Autodesk Fusion 360 part; units mm, degrees
(part 3 of 3)
ref_plane "WorkPlane14" through (0, 0, 17) normal (0, 0, 1) x (1, 0, 0)
sketch "Sketch18" plane through (0, 0, 17) normal (0, 0, 1) x (1, 0, 0)
  line L0 (575, 155) -> (300, 155)
  line L1 (575, 155) -> (575, 244.7658)
  line L2 (575, 244.7658) -> (300, 244.7658)
  line L3 (300, 244.7658) -> (300, 155)
  constraint horizontal L0
  constraint perpendicular L0 L1
  constraint perpendicular L1 L2
  constraint perpendicular L0 L3
extrude "Extrude17" cut sketch "Sketch18" against normal blind 200 bodies 6 7 8 9
extrude "Extrude18" add sketch "Sketch17" along normal mid plane 5 separate body makes body 13
mirror "Mirror2" about plane through (0, 0, 0) normal (1, 0, 0) of bodies 10 9 8 7 6 5 4 3 2 11 12 makes body 14 at (-72.5, 40.7662, 5.9313) makes body 15 at (-140, 40.7662, 5.9313) makes body 16 at (-211.5, 40.7662, 5.9313) makes body 17 at (-281.5, 40.7662, 5.9313) makes body 18 at (-351.5, 104.4646, 6.1744) makes body 19 at (-421.5, 104.4646, 6.1744) makes body 20 at (-491.5, 104.4646, 6.1744) makes body 21 at (-561.5, 104.4646, 6.1744) makes body 22 at (-600, 40.7662, 5.9313) makes body 23 at (-200, 62.2055, 10.1217) makes body 24 at (-200, 143.3882, 7.5489)
sketch "Sketch19" plane through (600, 0, 0) normal (1, 0, 0) x (0, 1, 0)
  spline S0 degree 3 poles (61.2364, 16.8866) (62.5517, 16.9377) (63.97, 16.9799) (65.4867, 17.0124) (69.0475, 17.0885) (73.1641, 17.1099) (77.299, 17.0516) (81.1898, 16.9968) (85.0421, 16.869) (88.6866, 16.6762) (93.5117, 16.421) (98.0281, 16.059) (102.6424, 15.6416) (107.4083, 15.2105) (112.3122, 14.7191) (117.3527, 14.1433) (123.7504, 13.4125) (130.3032, 12.5277) (136.4155, 11.5838) (140.28, 10.987) (143.9527, 10.3752) (147.6957, 9.7206) (151.3487, 9.0818) (155.1437, 8.3909) (159.2882, 7.6111) (162.7518, 6.9595) (166.4626, 6.2444) (170.0047, 5.5188) (173.5306, 4.7965) (176.8181, 4.0717) (179.5028, 3.4129) (180.7522, 3.1063) (181.8753, 2.8143) (182.9209, 2.533) knots 0 0 0 0 0.009474 0.009474 0.009474 0.031716 0.031716 0.031716 0.052644 0.052644 0.052644 0.080353 0.080353 0.080353 0.108972 0.108972 0.108972 0.145296 0.145296 0.145296 0.168261 0.168261 0.168261 0.190675 0.190675 0.190675 0.209405 0.209405 0.209405 0.22805 0.22805 0.22805 0.236727 0.236727 0.236727 0.236727
  spline S1 degree 3 poles (182.9209, 2.533) (181.6615, 2.4681) (180.2835, 2.4098) (178.7296, 2.3656) (175.4512, 2.2724) (171.3919, 2.2497) (167.2511, 2.2303) (163.72, 2.2137) (160.1948, 2.1893) (156.9225, 2.1285) (150.7153, 2.0131) (145.3748, 1.778) (139.6944, 1.5684) (135.7191, 1.4217) (131.5605, 1.2846) (127.3, 1.1404) (121.7528, 0.9526) (116.1156, 0.7389) (110.7376, 0.5168) (105.8624, 0.3155) (101.2103, 0.121) (96.4895, -0.064) (92.2873, -0.2286) (87.9529, -0.3939) (83.3434, -0.5864) (76.92, -0.8547) (69.9758, -1.181) (64.4566, -1.4428) (61.5509, -1.5807) (59.0608, -1.6981) (56.8136, -1.8047) (54.3796, -1.9201) (52.1544, -2.0283) (49.7746, -2.1475) (47.2437, -2.2742) (44.569, -2.411) (41.9726, -2.5266) (39.3288, -2.6442) (36.8126, -2.7357) (34.1902, -2.7985) (32.0483, -2.8498) (29.7799, -2.8851) (27.506, -2.8972) (24.9582, -2.9109) (22.493, -2.8895) (20.5139, -2.8297) (18.3654, -2.7647) (16.7453, -2.6714) (15.0921, -2.5644) (13.7433, -2.4772) (12.3486, -2.3624) (10.7983, -2.1313) (9.285, -1.9057) (7.6681, -1.5709) (6.571, -1.2759) (5.7621, -1.0583) (5.2684, -0.8846) (4.7124, -0.6375) (4.273, -0.4422) (3.7574, -0.176) (3.3872, 0.0837) (3.1943, 0.219) (3.0543, 0.3464) (2.9897, 0.42) knots 0.354921 0.354921 0.354921 0.354921 0.364912 0.364912 0.364912 0.385991 0.385991 0.385991 0.403967 0.403967 0.403967 0.438064 0.438064 0.438064 0.461927 0.461927 0.461927 0.492997 0.492997 0.492997 0.521162 0.521162 0.521162 0.546233 0.546233 0.546233 0.58117 0.58117 0.58117 0.599563 0.599563 0.599563 0.619485 0.619485 0.619485 0.640672 0.640672 0.640672 0.662246 0.662246 0.662246 0.679868 0.679868 0.679868 0.699613 0.699613 0.699613 0.721048 0.721048 0.721048 0.738537 0.738537 0.738537 0.755608 0.755608 0.755608 0.768195 0.768195 0.768195 0.778142 0.778142 0.778142 0.783322 0.783322 0.783322 0.783322
  spline S2 degree 3 poles (2.9897, 0.42) (3.0156, 0.5398) (3.1087, 0.7992) (3.2914, 1.117) (3.595, 1.6449) (4.1116, 2.2804) (4.5699, 2.7504) (5.0032, 3.1949) (5.3517, 3.4854) (5.6921, 3.7303) (6.0525, 3.9896) (6.4838, 4.2504) (7.1019, 4.6035) (7.8857, 5.0512) (8.9215, 5.6226) (9.9999, 6.1844) (11.2189, 6.8194) (12.4462, 7.4031) (13.5524, 7.8653) (15.2258, 8.5644) (16.6918, 9.0644) (18.3739, 9.632) (19.7064, 10.0816) (21.2216, 10.5662) (23.0631, 11.091) (25.1848, 11.6956) (27.6916, 12.3395) (30.1291, 12.901) (32.4156, 13.4278) (34.6015, 13.8747) (36.7294, 14.2509) (39.0596, 14.6628) (41.401, 15.0055) (43.8366, 15.324) (46.5535, 15.6792) (49.2932, 15.9964) (51.8513, 16.2482) (54.837, 16.5421) (57.6324, 16.7467) (61.2364, 16.8866) knots 0.79486 0.79486 0.79486 0.79486 0.800757 0.800757 0.800757 0.810556 0.810556 0.810556 0.819821 0.819821 0.819821 0.829628 0.829628 0.829628 0.842064 0.842064 0.842064 0.856122 0.856122 0.856122 0.877389 0.877389 0.877389 0.894237 0.894237 0.894237 0.913649 0.913649 0.913649 0.931858 0.931858 0.931858 0.951798 0.951798 0.951798 0.97404 0.97404 0.97404 1 1 1 1
  spline S3 degree 5 poles (61.12, 19.8844) (60.637, 19.8656) (59.6922, 19.8261) (58.3363, 19.7608) (56.6343, 19.6612) (54.619, 19.5144) (52.6451, 19.3434) (50.6512, 19.1472) (48.602, 18.9264) (46.5002, 18.6835) (44.3706, 18.4219) (42.246, 18.1437) (40.1536, 17.8487) (38.0987, 17.5329) (36.0579, 17.1875) (33.9968, 16.8029) (31.8851, 16.3717) (29.7097, 15.8913) (27.4942, 15.3676) (25.2995, 14.8155) (23.2007, 14.2542) (21.2669, 13.7028) (19.543, 13.177) (18.0246, 12.6838) (16.6574, 12.2197) (15.3629, 11.7682) (14.0587, 11.2993) (12.6796, 10.7659) (11.1943, 10.128) (9.6168, 9.3729) (8.0285, 8.5465) (6.5667, 7.749) (5.3418, 7.0607) (4.3846, 6.494) (3.5469, 5.9078) (2.6176, 5.0911) (1.5165, 3.9094) (0.4773, 2.4376) (-0.1465, 0.8714) (-0.0619, -0.564) (0.722, -1.7188) (1.8623, -2.5675) (2.9736, -3.1567) (3.9079, -3.575) (4.8464, -3.9155) (6.019, -4.2496) (7.4743, -4.59) (9.1101, -4.9106) (10.7731, -5.1743) (12.345, -5.3623) (13.7964, -5.4879) (15.1531, -5.5769) (16.4825, -5.6547) (17.8722, -5.7297) (19.4072, -5.799) (21.1491, -5.8545) (23.1072, -5.8903) (25.2368, -5.9054) (27.4654, -5.9014) (29.714, -5.8817) (31.9176, -5.8493) (34.0511, -5.8058) (36.1282, -5.7511) (38.181, -5.6845) (40.2457, -5.6055) (42.347, -5.5148) (44.4793, -5.4149) (46.615, -5.3099) (48.7209, -5.2041) (50.7726, -5.101) (52.7684, -5.0022) (54.7458, -4.9063) (56.7672, -4.8101) (58.9035, -4.7092) (61.2187, -4.5998) (63.7533, -4.4796) (66.5097, -4.3487) (69.462, -4.2092) (72.564, -4.0644) (75.7583, -3.9183) (78.985, -3.7745) (82.1901, -3.6364) (85.3351, -3.5056) (88.403, -3.3821) (91.3932, -3.2647) (94.3176, -3.1511) (97.1963, -3.039) (100.0533, -2.9259) (102.9129, -2.8103) (105.7944, -2.6913) (108.7102, -2.5697) (111.6664, -2.4469) (114.6637, -2.3247) (117.6975, -2.2052) (120.7588, -2.0898) (123.8347, -1.9795) (126.9085, -1.8739) (129.9619, -1.7717) (132.9775, -1.6708) (135.9416, -1.5694) (138.8471, -1.4658) (141.6962, -1.3598) (144.5027, -1.2521) (147.2962, -1.146) (150.117, -1.0461) (153.0074, -0.9575) (156.004, -0.8848) (159.1292, -0.8308) (162.3835, -0.7955) (165.7378, -0.7755) (169.123, -0.7621) (172.4448, -0.7441) (175.6031, -0.7098) (178.5092, -0.6507) (181.1051, -0.5633) (183.381, -0.4524) (185.3935, -0.3335) (187.2848, -0.2357) (189.2303, -0.1908) (191.3831, -0.2214) (193.8227, -0.3307) (196.496, -0.4891) (199.1776, -0.6277) (201.5529, -0.6648) (203.2912, -0.5318) (204.1194, -0.195) (203.9033, 0.3094) (202.699, 0.8841) (200.7124, 1.4729) (198.2365, 2.0427) (195.585, 2.582) (193.0295, 3.0932) (190.7296, 3.5872) (188.6853, 4.0776) (186.7958, 4.5791) (184.9056, 5.1048) (182.8532, 5.6644) (180.5234, 6.2618) (177.8817, 6.8932) (174.9494, 7.5502) (171.7902, 8.2207) (168.4917, 8.8914) (165.1491, 9.5491) (161.8488, 10.1828) (158.65, 10.7855) (155.5748, 11.3555) (152.6192, 11.8943) (149.7596, 12.4062) (146.96, 12.8967) (144.1802, 13.3716) (141.3828, 13.8358) (138.5414, 14.2923) (135.6441, 14.7413) (132.6897, 15.1815) (129.6857, 15.6102) (126.6452, 16.0244) (123.585, 16.421) (120.5226, 16.7977) (117.4739, 17.1533) (114.4514, 17.4884) (111.4639, 17.8039) (108.5159, 18.1017) (105.6069, 18.383) (102.7305, 18.6492) (99.8745, 18.9002) (97.0192, 19.1349) (94.1405, 19.3507) (91.2143, 19.5444) (88.221, 19.7125) (85.1491, 19.852) (82.0002, 19.9602) (78.7922, 20.0358) (75.5651, 20.0792) (72.3733, 20.092) (69.2771, 20.0768) (66.3336, 20.0363) (64.1373, 19.9858) (62.5903, 19.9386) (61.603, 19.9031) (61.12, 19.8844) knots -1 -1 -1 -1 -1 -1 -0.99428571 -0.98857143 -0.98285714 -0.97714286 -0.97142857 -0.96571429 -0.96 -0.95428571 -0.94857143 -0.94285714 -0.93714286 -0.93142857 -0.92571429 -0.92 -0.91428571 -0.90857143 -0.90285714 -0.89714286 -0.89142857 -0.88571429 -0.88 -0.87428571 -0.86857143 -0.86285714 -0.85714286 -0.85142857 -0.84571429 -0.84 -0.83428571 -0.82857143 -0.82285714 -0.81714286 -0.81142857 -0.80571429 -0.8 -0.79428571 -0.78857143 -0.78285714 -0.77714286 -0.77142857 -0.76571429 -0.76 -0.75428571 -0.74857143 -0.74285714 -0.73714286 -0.73142857 -0.72571429 -0.72 -0.71428571 -0.70857143 -0.70285714 -0.69714286 -0.69142857 -0.68571429 -0.68 -0.67428571 -0.66857143 -0.66285714 -0.65714286 -0.65142857 -0.64571429 -0.64 -0.63428571 -0.62857143 -0.62285714 -0.61714286 -0.61142857 -0.60571429 -0.6 -0.59428571 -0.58857143 -0.58285714 -0.57714286 -0.57142857 -0.56571429 -0.56 -0.55428571 -0.54857143 -0.54285714 -0.53714286 -0.53142857 -0.52571429 -0.52 -0.51428571 -0.50857143 -0.50285714 -0.49714286 -0.49142857 -0.48571429 -0.48 -0.47428571 -0.46857143 -0.46285714 -0.45714286 -0.45142857 -0.44571429 -0.44 -0.43428571 -0.42857143 -0.42285714 -0.41714286 -0.41142857 -0.40571429 -0.4 -0.39428571 -0.38857143 -0.38285714 -0.37714286 -0.37142857 -0.36571429 -0.36 -0.35428571 -0.34857143 -0.34285714 -0.33714286 -0.33142857 -0.32571429 -0.32 -0.31428571 -0.30857143 -0.30285714 -0.29714286 -0.29142857 -0.28571429 -0.28 -0.27428571 -0.26857143 -0.26285714 -0.25714286 -0.25142857 -0.24571429 -0.24 -0.23428571 -0.22857143 -0.22285714 -0.21714286 -0.21142857 -0.20571429 -0.2 -0.19428571 -0.18857143 -0.18285714 -0.17714286 -0.17142857 -0.16571429 -0.16 -0.15428571 -0.14857143 -0.14285714 -0.13714286 -0.13142857 -0.12571429 -0.12 -0.11428571 -0.10857143 -0.10285714 -0.09714286 -0.09142857 -0.08571429 -0.08 -0.07428571 -0.06857143 -0.06285714 -0.05714286 -0.05142857 -0.04571429 -0.04 -0.03428571 -0.02857143 -0.02285714 -0.01714286 -0.01142857 -0.00571429 0 0 0 0 0 0
  circle A0 centre (177.9946, 6.8231) radius 0.025
  dimension "d85" = 0.05
  measures "d85" diameter of A0
extrude "Extrude19" add sketch "Sketch19" against normal blind 600 separate body contours A0 makes body 25
ref_plane "WorkPlane15" through (600, 177.9782, 6.8605) normal (0, 0.226022, 0.974122) x (-1, 0, 0)
sketch "Sketch20" plane through (0, 10.6027, 45.6961) normal (0, 0.226022, 0.974122) x (-1, 0, 0)
  line L0 (-301, -150.9889) -> (-599, -150.9889)
  line L1 (-301, -194.8244) -> (-301, -150.9889)
  line L2 (-599, -194.8244) -> (-301, -194.8244)
  line L3 (-599, -150.9889) -> (-599, -194.8244)
  line L4 (599, -194.8244) -> (301, -194.8244)
  line L5 (301, -150.9889) -> (599, -150.9889)
  line L6 (301, -194.8244) -> (301, -150.9889)
  line L7 (599, -150.9889) -> (599, -194.8244)
extrude "Extrude20" add sketch "Sketch20" against normal blind 2.5 separate body contours L0 L1 L2 L3 makes body 26
mirror "Mirror3" about plane through (0, 0, 0) normal (1, 0, 0) of bodies 26 makes body 27
ref_plane "WorkPlane16" through (600, 0, 0) normal (1, 0, 0) x (0, 1, 0)
sketch "Sketch21" plane through (600, 0, 0) normal (1, 0, 0) x (0, 1, 0)
  spline S0 degree 3 poles (2.9897, 0.42) (3.0543, 0.3464) (3.1943, 0.219) (3.3872, 0.0837) (3.7574, -0.176) (4.273, -0.4422) (4.7124, -0.6375) (5.2684, -0.8846) (5.7621, -1.0583) (6.571, -1.2759) (7.6681, -1.5709) (9.285, -1.9057) (10.7983, -2.1313) (12.3486, -2.3624) (13.7433, -2.4772) (15.0921, -2.5644) (16.7453, -2.6714) (18.3654, -2.7647) (20.5139, -2.8297) (22.493, -2.8895) (24.9582, -2.9109) (27.506, -2.8972) (29.7799, -2.8851) (32.0483, -2.8498) (34.1902, -2.7985) (36.8126, -2.7357) (39.3288, -2.6442) (41.9726, -2.5266) (44.569, -2.411) (47.2437, -2.2742) (49.7746, -2.1475) (52.1544, -2.0283) (54.3796, -1.9201) (56.8136, -1.8047) (59.0608, -1.6981) (61.5509, -1.5807) (64.4566, -1.4428) (69.9758, -1.181) (76.92, -0.8547) (83.3434, -0.5864) (87.9529, -0.3939) (92.2873, -0.2286) (96.4895, -0.064) (101.2103, 0.121) (105.8624, 0.3155) (110.7376, 0.5168) (116.1156, 0.7389) (121.7528, 0.9526) (127.3, 1.1404) (131.5605, 1.2846) (135.7191, 1.4217) (139.6944, 1.5684) (145.3748, 1.778) (150.7153, 2.0131) (156.9225, 2.1285) (160.1948, 2.1893) (163.72, 2.2137) (167.2511, 2.2303) (171.3919, 2.2497) (175.4512, 2.2724) (178.7296, 2.3656) (180.2835, 2.4098) (181.6615, 2.4681) (182.9209, 2.533) knots -0.783322 -0.783322 -0.783322 -0.783322 -0.778142 -0.778142 -0.778142 -0.768195 -0.768195 -0.768195 -0.755608 -0.755608 -0.755608 -0.738537 -0.738537 -0.738537 -0.721048 -0.721048 -0.721048 -0.699613 -0.699613 -0.699613 -0.679868 -0.679868 -0.679868 -0.662246 -0.662246 -0.662246 -0.640672 -0.640672 -0.640672 -0.619485 -0.619485 -0.619485 -0.599563 -0.599563 -0.599563 -0.58117 -0.58117 -0.58117 -0.546233 -0.546233 -0.546233 -0.521162 -0.521162 -0.521162 -0.492997 -0.492997 -0.492997 -0.461927 -0.461927 -0.461927 -0.438064 -0.438064 -0.438064 -0.403967 -0.403967 -0.403967 -0.385991 -0.385991 -0.385991 -0.364912 -0.364912 -0.364912 -0.354921 -0.354921 -0.354921 -0.354921
  spline S1 degree 3 poles (182.9209, 2.533) (181.8753, 2.8143) (180.7522, 3.1063) (179.5028, 3.4129) (176.8181, 4.0717) (173.5306, 4.7965) (170.0047, 5.5188) (166.4626, 6.2444) (162.7518, 6.9595) (159.2882, 7.6111) (155.1437, 8.3909) (151.3487, 9.0818) (147.6957, 9.7206) (143.9527, 10.3752) (140.28, 10.987) (136.4155, 11.5838) (130.3032, 12.5277) (123.7504, 13.4125) (117.3527, 14.1433) (112.3122, 14.7191) (107.4083, 15.2105) (102.6424, 15.6416) (98.0281, 16.059) (93.5117, 16.421) (88.6866, 16.6762) (85.0421, 16.869) (81.1898, 16.9968) (77.299, 17.0516) (73.1641, 17.1099) (69.0475, 17.0885) (65.4867, 17.0124) (63.97, 16.9799) (62.5517, 16.9377) (61.2364, 16.8866) knots -0.236727 -0.236727 -0.236727 -0.236727 -0.22805 -0.22805 -0.22805 -0.209405 -0.209405 -0.209405 -0.190675 -0.190675 -0.190675 -0.168261 -0.168261 -0.168261 -0.145296 -0.145296 -0.145296 -0.108972 -0.108972 -0.108972 -0.080353 -0.080353 -0.080353 -0.052644 -0.052644 -0.052644 -0.031716 -0.031716 -0.031716 -0.009474 -0.009474 -0.009474 0 0 0 0
  spline S2 degree 3 poles (61.2364, 16.8866) (57.6324, 16.7467) (54.837, 16.5421) (51.8513, 16.2482) (49.2932, 15.9964) (46.5535, 15.6792) (43.8366, 15.324) (41.401, 15.0055) (39.0596, 14.6628) (36.7294, 14.2509) (34.6015, 13.8747) (32.4156, 13.4278) (30.1291, 12.901) (27.6916, 12.3395) (25.1848, 11.6956) (23.0631, 11.091) (21.2216, 10.5662) (19.7064, 10.0816) (18.3739, 9.632) (16.6918, 9.0644) (15.2258, 8.5644) (13.5524, 7.8653) (12.4462, 7.4031) (11.2189, 6.8194) (9.9999, 6.1844) (8.9215, 5.6226) (7.8857, 5.0512) (7.1019, 4.6035) (6.4838, 4.2504) (6.0525, 3.9896) (5.6921, 3.7303) (5.3517, 3.4854) (5.0032, 3.1949) (4.5699, 2.7504) (4.1116, 2.2804) (3.595, 1.6449) (3.2914, 1.117) (3.1087, 0.7992) (3.0156, 0.5398) (2.9897, 0.42) knots -1 -1 -1 -1 -0.97404 -0.97404 -0.97404 -0.951798 -0.951798 -0.951798 -0.931858 -0.931858 -0.931858 -0.913649 -0.913649 -0.913649 -0.894237 -0.894237 -0.894237 -0.877389 -0.877389 -0.877389 -0.856122 -0.856122 -0.856122 -0.842064 -0.842064 -0.842064 -0.829628 -0.829628 -0.829628 -0.819821 -0.819821 -0.819821 -0.810556 -0.810556 -0.810556 -0.800757 -0.800757 -0.800757 -0.79486 -0.79486 -0.79486 -0.79486
  line L0 (2.9897, 0.42) -> (182.9209, 2.533) construction
  line L1 (92.9553, 1.4765) -> (92.7797, 16.4307) construction
  line L2 (92.9553, 1.4765) -> (92.975, -0.201) construction
  point P0 (92.8773, 8.1148)
  constraint coincident S0.start S2.end
  constraint coincident S0.end S1.start
  constraint midpoint L0 L1.start
  constraint coincident S1 L1.end
  constraint perpendicular L0 L1
  constraint coincident S0 L2.end
  constraint perpendicular L0 L2
extrude "Extrude21" add sketch "Sketch21" along normal blind 3 separate body makes body 28
extrude "Extrude22" add sketch "Sketch21" along normal blind 3 separate body makes body 29
scale "Scale1" factor 1.5 about (600, 92.8773, 8.1148) bodies 28
mirror "Mirror4" about plane through (0, 0, 0) normal (1, 0, 0) of bodies 28 makes body 30
